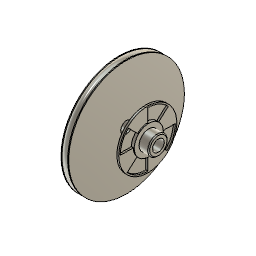
プーリー＆センサスリット (Autodesk Fusion 360 design; units mm, degrees)
Autodesk Fusion 360 part; units mm, degrees
note: some values were not read from the file. Set by a fixed rule: which sketch regions a step uses.
sketch "スケッチ1" plane through (0, 0, 0) normal (0, 0, 1) x (1, 0, 0)
  circle A0 centre (0, 0) radius 30
  circle A1 centre (0, 0) radius 6
  circle A2 centre (0, 0) radius 28.5
  circle A3 centre (0, 0) radius 10
  line L0 (0, -10) -> (0, -28.5)
  line L1 (10, 0) -> (28.5, 0)
  line L2 (0, 10) -> (0, 28.5)
  line L3 (-10, 0) -> (-28.5, 0)
  line L4 (0, 28.5) -> (28.5, 0)
  line L5 (14.25, 14.25) -> (20.1525, 20.1525)
  line L6 (20.1525, 20.1525) -> (0, 0)
  line L7 (0, 0) -> (-21.2132, -21.2132)
  line L8 (0, 0) -> (19.0329, -21.2132)
  line L9 (0, 0) -> (-19.0329, 21.2132)
  dimension "d1" = 60
  dimension "d2" = 12
  dimension "d3" = 57
  dimension "d5" = 360
  constraint coincident A0.centre A1.centre
  constraint concentric A0 A2
  constraint concentric A2 A3
  constraint coincident A2 L0.end
  constraint coincident A3 L0.start
  constraint midpoint L4 L5.start
  constraint coincident A2 L5.end
  constraint perpendicular L4 L5
  constraint coincident A0 L7.end
  constraint parallel L6 L7
  constraint coincident A2 L8.end
  constraint coincident A2 L9.end
  constraint parallel L8 L9
  measures "d1" diameter of A0
  measures "d2" diameter of A1
  measures "d3" diameter of A2
extrude "押し出し1" add sketch "スケッチ1" along normal blind 2 contours A0 | A3 L1 L4 L6 | A2 A3 L0 L8 | A2 A3 L2 L9 | A2 L4 L5 L6 | A2 A3 L3 L7 picked at (19.0044, 17.2507) makes body 1
sketch "スケッチ2" plane through (0, 0, 0) normal (0, 0, 1) x (1, 0, 0)
  circle A0 centre (0, 0) radius 15
  circle A1 centre (0, 0) radius 6
  circle A2 centre (0, 0) radius 6
  constraint coincident A0.centre A1.centre
  constraint concentric A0 A2
extrude "押し出し2" add sketch "スケッチ2" along normal blind 3 bodies 1
sketch "スケッチ3" plane through (0, 0, 3) normal (0, 0, 1) x (-1, 0, 0)
  circle A0 centre (0, 0) radius 30
  circle A1 centre (0, 0) radius 10
  line L0 (0, 15) -> (0, 28.5)
  arc A2 (19.0329, -21.2132) -> (28.5, 0) centre (0, 0) ccw
  line L1 (15, 0) -> (28.5, 0)
  arc A3 (0, -15) -> (10.0173, -11.1648) centre (0, 0) ccw
  line L2 (0, -15) -> (0, -28.5)
  line L3 (-15, 0) -> (-28.5, 0)
  circle A4 centre (0, 0) radius 6
  arc A5 (-20.1525, -20.1525) -> (0, -28.5) centre (0, 0) ccw
  line L4 (-20.1525, -20.1525) -> (-10.6066, -10.6066)
  arc A6 (-15, 0) -> (-10.6066, -10.6066) centre (0, 0) ccw
  arc A7 (-19.0329, 21.2132) -> (-28.5, 0) centre (0, 0) ccw
  line L5 (-19.0329, 21.2132) -> (-10.0173, 11.1648)
  arc A8 (0, 15) -> (-10.0173, 11.1648) centre (0, 0) ccw
  arc A9 (20.1525, 20.1525) -> (0, 28.5) centre (0, 0) ccw
  line L6 (20.1525, 20.1525) -> (10.6066, 10.6066)
  arc A10 (15, 0) -> (10.6066, 10.6066) centre (0, 0) ccw
  line L7 (19.0329, -21.2132) -> (10.0173, -11.1648)
  constraint concentric A0 A4
extrude "押し出し3" add sketch "スケッチ3" along normal blind 10 contours A1 bodies 1
chamfer "面取り1" distance 1 angle 45 1 edges at (9.3233, 3.6162, 13) on bodies 1
sketch "スケッチ4" plane through (0, 0, 0) normal (1, 0, 0) x (0, 1, 0)
  line L0 (0, 3) -> (0, 6)
  constraint vertical L0
sketch "スケッチ5" plane through (0, 0, 0) normal (0, 0, 1) x (1, 0, 0)
sketch "スケッチ6" plane through (0, 0, 0) normal (0, 0, 1) x (1, 0, 0)
  circle A0 centre (-75, 0) radius 15
  circle A1 centre (-75, 0) radius 6
  dimension "d16" = 12
  constraint concentric A0 A1
  measures "d16" diameter of A1
sketch "スケッチ8" plane through (0, 0, 0) normal (0, 1, 0) x (1, 0, 0)
  circle A0 centre (-90, -4) radius 2.75
  line L0 (-75, 0) -> (-75, -16)
  dimension "d21" = 5.5
  constraint vertical L0
  measures "d21" diameter of A0
sketch "スケッチ9" plane through (0, 0, 0) normal (0, 0, 1) x (1, 0, 0)
  circle A0 centre (-120, 0) radius 15
  circle A1 centre (-120, 0) radius 1.05
  dimension "d25" = 2.1
  constraint concentric A0 A1
  measures "d25" diameter of A1
extrude "押し出し6" add sketch "スケッチ9" along normal blind 8 separate body makes body 2
sketch "スケッチ10" plane through (0, 0, 0) normal (0, 1, 0) x (1, 0, 0)
  line L0 (-120, 0) -> (-120, -10)
  circle A0 centre (-135, -4) radius 2.75
  dimension "d28" = 5.5
  constraint vertical L0
  measures "d28" diameter of A0
revolve "回転2" cut sketch "スケッチ10" angle 360 about axis through (-120, 0, 0) along (0, 0, 1) bodies 2
sketch "スケッチ11" plane through (0, 0, 0) normal (0, 0, 1) x (1, 0, 0)
  line L0 (0, 50) -> (60, 50)
  line L1 (60, 50) -> (60, 59)
  line L2 (60, 59) -> (0, 59)
  line L3 (0, 59) -> (0, 50)
  dimension "d30" = 60
  dimension "d31" = 9
  constraint horizontal L0
  constraint vertical L1
  constraint horizontal L2
  constraint vertical L3
  measures "d30" distance of L0.start L0.end
  measures "d31" distance of L0.start L2.end
sketch "スケッチ14" plane through (0, 0, 0) normal (0, 0, 1) x (1, 0, 0)
  line L0 (60, 60) -> (-65, 60)
  line L1 (-65, 60) -> (-65, 125)
  line L2 (-65, 125) -> (60, 125)
  line L3 (60, 125) -> (60, 60)
  dimension "d45" = 125
  dimension "d46" = 65
  constraint horizontal L0
  constraint vertical L1
  constraint horizontal L2
  constraint vertical L3
  measures "d45" distance of L0.start L0.end
  measures "d46" distance of L0.start L2.end
sketch "スケッチ15" plane through (0, 0, 0) normal (0, 0, 1) x (1, 0, 0)
sketch "スケッチ21" plane through (0, 0, 0) normal (0, 0, 1) x (1, 0, 0)
  circle A0 centre (100, 0) radius 60
  circle A1 centre (100, 0) radius 6
  dimension "d69" = 120
  dimension "d70" = 12
  constraint concentric A0 A1
  measures "d69" diameter of A0
  measures "d70" diameter of A1
extrude "押し出し12" add sketch "スケッチ21" along normal blind 8 separate body makes body 3
sketch "スケッチ22" plane through (0, 0, 8) normal (0, 0, 1) x (-1, 0, 0)
  circle A0 centre (-100, 0) radius 6
  circle A1 centre (-100, 0) radius 60
  circle A2 centre (-100, 0) radius 10
  dimension "d73" = 20
  constraint concentric A0 A2
  measures "d73" diameter of A2
extrude "押し出し13" add sketch "スケッチ22" along normal blind 10 contours A2 bodies 3
chamfer "面取り6" distance 1 angle 45 1 edges at (109.3233, 3.6162, 18) on bodies 3
sketch "スケッチ23" plane through (0, 0, 0) normal (0, 1, 0) x (1, 0, 0)
  line L0 (100, -20) -> (100, 0)
  circle A0 centre (160, -4) radius 3
  constraint vertical L0
revolve "回転3" cut sketch "スケッチ23" angle 360 about axis through (100, 0, 20) along (0, 0, -1) bodies 3
sketch "スケッチ24" plane through (0, 0, 0) normal (0, 1, 0) x (1, 0, 0)
  line L0 (0, -13) -> (0, -8)
  line L1 (-75, -18) -> (-75, -13)
  line L2 (100, -18) -> (100, -13)
  point P0 (0, -8)
  point P1 (-75, -13)
  point P2 (100, -13)
  dimension "d78" = 5
  dimension "d79" = 5
  dimension "d80" = 5
  constraint vertical L0
  constraint coincident P0 L0.end
  constraint vertical L1
  constraint coincident P1 L1.end
  constraint vertical L2
  constraint coincident P2 L2.end
  measures "d78" distance of L0.start P0
  measures "d79" distance of L1.start P1
  measures "d80" distance of L2.start P2
move_body "移動1" bodies 2 to x (1, 0, 0) y (0, 1, 0) z (0, 0, 1) at (65, 0, 0)
move_body "移動2" bodies 1 to x (0, 0, -1) y (0, 1, 0) z (1, 0, 0) at (-30, 0, 0)
move_body "移動3" bodies 3 to x (0, 0, 1) y (0, 1, 0) z (-1, 0, 0) at (-50, 0, -100)
move_body "移動4" bodies 2 to x (0, 0, -1) y (0, 1, 0) z (1, 0, 0) at (-80, 0, -55)
named bodies: "センサスリット", "モータープーリー", "ピックアッププーリー"
